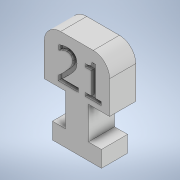
# Autodesk Inventor part: 2번부품
Saved by Autodesk Inventor 2022 (Build 260153000, 153)
## iProperties
Created: 2021-09-04
Part Number: 2번부품
Material: 일반
Document SubType Name: Modeling
Designer: 서울공업고등학교
Density: 1 g/cm^3
Appearance: 기본값
Author: 서울공업고등학교
Autodesk Inventor part; units mm, degrees
ref_plane "YZ Plane" through (0, 0, 0) normal (1, 0, 0) x (0, 1, 0)
ref_plane "XZ Plane" through (0, 0, 0) normal (0, 1, 0) x (-1, 0, 0)
ref_plane "XY Plane" through (0, 0, 0) normal (0, 0, 1) x (1, 0, 0)
sketch "스케치1" plane through (0, 0, 0) normal (0, 0, 1) x (1, 0, 0)
  line L0 (0, 0) -> (-10, 0)
  line L1 (-10, 0) -> (-10, -15)
  line L2 (-10, -15) -> (-3.5, -15)
  line L3 (-3.5, -15) -> (-3.5, -25)
  line L4 (-3.5, -25) -> (-7.5, -25)
  line L5 (-7.5, -25) -> (-7.5, -30)
  line L6 (-7.5, -30) -> (0, -30)
  line L7 (0, 0) -> (0, -30)
  dimension "d0" = 10
  dimension "d1" = 15
  dimension "d2" = 10
  dimension "d3" = 5
  dimension "d4" = 7.5
  dimension "d12" = 3.5
  constraints: 16 end point, 6 perpendicular, 1 horizontal
  measures "d0" distance of L0.start L0.end
  measures "d1" distance of L0.end L1.end
  measures "d2" distance of L2.end L3.end
  measures "d3" distance of L4.end L5.end
  measures "d4" distance of L5.end L6.end
  measures "d12" distance between parallel lines of L7 L3
extrude "돌출1" add sketch "스케치1" along normal mid plane 8
mirror "미러1" about plane through (0, 0, 0) normal (1, 0, 0) of "돌출1"
fillet "모깎기1" radius 5 2 edges at (10, 0, 0) (-10, 0, 0)
sketch "스케치2" plane through (0, 0, 4) normal (0, 0, 1) x (1, 0, 0)
  line L0 (-6.452, -3.1686) -> (7.8296, -3.1686) construction
  line L1 (7.8296, -3.1686) -> (7.8296, -13.9142) construction
  line L2 (7.8296, -13.9142) -> (-6.452, -13.9142) construction
  line L3 (-6.452, -13.9142) -> (-6.452, -3.1686) construction
  line L4 (0.4443, -13.3793) -> (-5.7226, -13.3793)
  line L5 (-5.7226, -13.3793) -> (-5.7226, -11.9611)
  spline S0 degree 2 poles (-5.7226, -11.9611) (-5.0581, -11.3371) (-3.875, -10.1783) (-3.3077, -9.5543) knots 0 0 0 1 2 2 2
  spline S1 degree 2 poles (-3.3077, -9.5543) (-2.1651, -8.2982) (-1.3304, -6.7909) (-1.3304, -5.9887) knots 0 0 0 1 2 2 2
  spline S2 degree 2 poles (-1.3304, -5.9887) (-1.3304, -5.5673) (-1.5897, -4.9352) (-1.8247, -4.7326) knots 0 0 0 1 2 2 2
  spline S3 degree 2 poles (-1.8247, -4.7326) (-2.0597, -4.53) (-2.6756, -4.3274) (-3.0484, -4.3274) knots 0 0 0 1 2 2 2
  spline S4 degree 2 poles (-3.0484, -4.3274) (-3.405, -4.3274) (-4.1343, -4.5057) (-4.4665, -4.6435) knots 0 0 0 1 2 2 2
  spline S5 degree 2 poles (-4.4665, -4.6435) (-4.7502, -4.7569) (-5.2769, -5.0811) (-5.439, -5.1945) knots 0 0 0 1 2 2 2
  line L6 (-5.439, -5.1945) -> (-5.5119, -5.1945)
  line L7 (-5.5119, -5.1945) -> (-5.5119, -3.7683)
  spline S6 degree 2 poles (-5.5119, -3.7683) (-5.0986, -3.5657) (-3.6157, -3.1686) (-2.9511, -3.1686) knots 0 0 0 1 2 2 2
  spline S7 degree 2 poles (-2.9511, -3.1686) (-1.5492, -3.1686) (0.031, -4.6516) (0.031, -5.9157) knots 0 0 0 1 2 2 2
  spline S8 degree 2 poles (0.031, -5.9157) (0.031, -6.5073) (-0.2445, -7.496) (-0.4876, -7.9174) knots 0 0 0 1 2 2 2
  spline S9 degree 2 poles (-0.4876, -7.9174) (-0.7307, -8.355) (-1.4358, -9.214) (-1.8247, -9.6272) knots 0 0 0 1 2 2 2
  spline S10 degree 2 poles (-1.8247, -9.6272) (-2.4568, -10.3161) (-4.0046, -11.7909) (-4.4665, -12.2204) knots 0 0 0 1 2 2 2
  line L8 (-4.4665, -12.2204) -> (0.4443, -12.2204)
  line L9 (0.4443, -12.2204) -> (0.4443, -13.3793)
  line L10 (7.4459, -13.3793) -> (2.5675, -13.3793)
  line L11 (2.5675, -13.3793) -> (2.5675, -12.3582)
  line L12 (2.5675, -12.3582) -> (4.3827, -12.3582)
  line L13 (4.3827, -12.3582) -> (4.3827, -5.6564)
  line L14 (4.3827, -5.6564) -> (2.5675, -5.6564)
  line L15 (2.5675, -5.6564) -> (2.5675, -4.7407)
  spline S11 degree 2 poles (2.5675, -4.7407) (3.5967, -4.7407) (4.5691, -4.1572) (4.6339, -3.3469) knots 0 0 0 1 2 2 2
  line L16 (4.6339, -3.3469) -> (5.6712, -3.3469)
  line L17 (5.6712, -3.3469) -> (5.6712, -12.3582)
  line L18 (5.6712, -12.3582) -> (7.4459, -12.3582)
  line L19 (7.4459, -12.3582) -> (7.4459, -13.3793)
  point P0 (0, 0)
  constraints: 2 other
extrude "돌출2" cut sketch "스케치2" against normal blind 1
